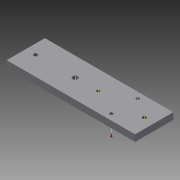
# Autodesk Inventor part: suport maneta vid
Saved by Autodesk Inventor 2015 SP1 (Build 190203100, 203)
## iProperties
Created: 2015-08-09
Part Number: suport maneta vid
Material: Generic
Document SubType Name: Modeling
Designer: ubik
Density: 1 g/cm^3
Appearance: Default
Author: ubik
Autodesk Inventor part; units mm, degrees
ref_plane "YZ Plane" through (0, 0, 0) normal (1, 0, 0) x (0, 1, 0)
ref_plane "XZ Plane" through (0, 0, 0) normal (0, 1, 0) x (-1, 0, 0)
ref_plane "XY Plane" through (0, 0, 0) normal (0, 0, 1) x (1, 0, 0)
sketch "Sketch1" plane through (0, 0, 0) normal (0, 0, 1) x (1, 0, 0)
  line L0 (-57.5, 29) -> (57.5, 29)
  line L1 (57.5, 29) -> (57.5, -29)
  line L2 (57.5, -29) -> (-57.5, -29)
  line L3 (-57.5, -29) -> (-57.5, 29)
  circle A0 centre (12.5, 0) radius 2.5
  circle A1 centre (52.5, 20) radius 2.5
  circle A2 centre (52.5, -20) radius 2.5
  circle A3 centre (-22.5, 0) radius 4
  point P0 (0, 0)
  dimension "d0" = 115
  dimension "d1" = 58
  dimension "d2" = 29
  dimension "d3" = 57.5
  dimension "d4" = 5
  dimension "d5" = 45
  dimension "d6" = 29
  dimension "d7" = 5
  dimension "d8" = 5
  dimension "d9" = 5
  dimension "d11" = 5
  dimension "d13" = 8
  dimension "d14" = 80
  dimension "d15" = 29
  dimension "d18" = 40
  dimension "d19" = 20
  dimension "d20" = 20
  constraints: 8 end point, 4 centre point, 2 parallel, 1 horizontal, 1 perpendicular
  measures "d0" distance of L1.end L2.end
  measures "d1" distance of L0.end L1.end
  measures "d2" distance from line of point (0, 0) L0
  measures "d3" distance from line of point (0, 0) L3
  measures "d4" diameter of A0
  measures "d5" distance from line of L1 A0.centre
  measures "d6" distance from line of L2 A0.centre
  measures "d7" diameter of A1
  measures "d8" diameter of A2
  measures "d9" distance from line of L1 A1.centre
  measures "d11" distance from line of L1 A2.centre
  measures "d13" diameter of A3
  measures "d14" distance from line of L1 A3.centre
  measures "d15" distance from line of L2 A3.centre
  measures "d18" distance of A1.centre A2.centre
  measures "d19" vertical distance of A0.centre A2.centre
  measures "d20" vertical distance of A0.centre A1.centre
extrude "Extrusion1" add sketch "Sketch1" along normal blind 10
sketch "Sketch3" plane through (-57.5, -29, 0) normal (-1, 0, 0) x (0, 0, 1)
  line L0 (0, 0) -> (0, 58) projected
  line L1 (0, 0) -> (10, 0) projected
  line L2 (10, 58) -> (10, 0) projected
  line L3 (0, 58) -> (10, 58) projected
  point P0 (0, 29)
extrude "Extrusion2" add sketch "Sketch3" along normal blind 40
sketch "Sketch4" plane through (57.5, -29, 0) normal (1, 0, 0) x (0, 0, -1)
  line L0 (0, 58) -> (0, 0) projected
  line L1 (0, 58) -> (-10, 58) projected
  line L2 (-10, 0) -> (-10, 58) projected
  line L3 (0, 0) -> (-10, 0) projected
  point P0 (0, 29)
extrude "Extrusion3" add sketch "Sketch4" along normal blind 40
hole "Hole1" at (82.5, 0, 0) direction (0, 0, 1) diameter 6 end through all counterbore diameter 10 counterbore depth 3
hole "Hole2" at (-82.5, 0, 0) direction (0, 0, 1) diameter 6 end through all counterbore diameter 10 counterbore depth 3
equation "\"d2\" = 0.5 * d1"
equation "\"d3\" = 0.5 * d0"
equation "\"d6\" = 0.5 * d1"
equation "\"d11\" = d9"
equation "\"d15\" = 0.5 * d1"
body "Solid1"
